Autodesk Fusion 360 part; units mm, degrees
note: some values were not read from the file. Set by a fixed rule: which face or edge a step refers to.
(part 2 of 2)
sketch "Skizze8" plane through (0, 0, 66) normal (0, 0, -1) x (-1, 0, 0)
  circle A0 centre (6.1, 44.01) radius 2
  line L0 (-43.85, 38.01) -> (0.1, 38.01)
  line L1 (0.1, 38.01) -> (0.1, -0.01)
  line L2 (0.1, -0.01) -> (-43.85, -0.01)
  line L3 (-43.85, -0.01) -> (-43.85, 38.01)
  circle A1 centre (-49.85, -6.01) radius 2
  circle A2 centre (-49.85, 44.01) radius 2
  circle A3 centre (6.1, -6.01) radius 2
  arc A4 (-49.85, 48.01) -> (-53.85, 44.01) centre (-49.85, 44.01) ccw
  line L4 (-53.85, 44.01) -> (-53.85, -6.01)
  arc A5 (-53.85, -6.01) -> (-49.85, -10.01) centre (-49.85, -6.01) ccw
  line L5 (-49.85, -10.01) -> (6.1, -10.01)
  arc A6 (6.1, -10.01) -> (10.1, -6.01) centre (6.1, -6.01) ccw
  line L6 (10.1, -6.01) -> (10.1, 44.01)
  arc A7 (10.1, 44.01) -> (6.1, 48.01) centre (6.1, 44.01) ccw
  line L7 (6.1, 48.01) -> (-49.85, 48.01)
  line L8 (0.1, -0.01) -> (-43.85, -0.01)
  line L9 (-43.85, -0.01) -> (-43.85, 38.01)
  line L10 (-43.85, 38.01) -> (0.1, 38.01)
  line L11 (0.1, 38.01) -> (0.1, -0.01)
  line L12 (-43.85, 38.01) -> (0.1, 38.01)
  line L13 (0.1, 38.01) -> (0.1, 38)
  line L14 (0.1, 38) -> (-43.85, 38)
  line L15 (-43.85, 38) -> (-43.85, 38.01)
  line L16 (-43.85, 0) -> (0.1, 0)
  line L17 (0.1, 0) -> (0.1, -0.01)
  line L18 (0.1, -0.01) -> (-43.85, -0.01)
  line L19 (-43.85, -0.01) -> (-43.85, 0)
  line L20 (-43.85, 2) -> (0.1, 2)
  line L21 (0.1, 2) -> (0.1, 0)
  line L22 (0.1, 0) -> (-43.85, 0)
  line L23 (-43.85, 0) -> (-43.85, 2)
  line L24 (-43.85, 4) -> (0.1, 4)
  line L25 (0.1, 4) -> (0.1, 2)
  line L26 (0.1, 2) -> (-43.85, 2)
  line L27 (-43.85, 2) -> (-43.85, 4)
  line L28 (-43.85, 6) -> (0.1, 6)
  line L29 (0.1, 6) -> (0.1, 4)
  line L30 (0.1, 4) -> (-43.85, 4)
  line L31 (-43.85, 4) -> (-43.85, 6)
  line L32 (-43.85, 8) -> (0.1, 8)
  line L33 (0.1, 8) -> (0.1, 6)
  line L34 (0.1, 6) -> (-43.85, 6)
  line L35 (-43.85, 6) -> (-43.85, 8)
  line L36 (-43.85, 10) -> (0.1, 10)
  line L37 (0.1, 10) -> (0.1, 8)
  line L38 (0.1, 8) -> (-43.85, 8)
  line L39 (-43.85, 8) -> (-43.85, 10)
  line L40 (-43.85, 12) -> (0.1, 12)
  line L41 (0.1, 12) -> (0.1, 10)
  line L42 (0.1, 10) -> (-43.85, 10)
  line L43 (-43.85, 10) -> (-43.85, 12)
  line L44 (-43.85, 14) -> (0.1, 14)
  line L45 (0.1, 14) -> (0.1, 12)
  line L46 (0.1, 12) -> (-43.85, 12)
  line L47 (-43.85, 12) -> (-43.85, 14)
  line L48 (-43.85, 16) -> (0.1, 16)
  line L49 (0.1, 16) -> (0.1, 14)
  line L50 (0.1, 14) -> (-43.85, 14)
  line L51 (-43.85, 14) -> (-43.85, 16)
  line L52 (-43.85, 18) -> (0.1, 18)
  line L53 (0.1, 18) -> (0.1, 16)
  line L54 (0.1, 16) -> (-43.85, 16)
  line L55 (-43.85, 16) -> (-43.85, 18)
  line L56 (-43.85, 20) -> (0.1, 20)
  line L57 (0.1, 20) -> (0.1, 18)
  line L58 (0.1, 18) -> (-43.85, 18)
  line L59 (-43.85, 18) -> (-43.85, 20)
  line L60 (-43.85, 22) -> (0.1, 22)
  line L61 (0.1, 22) -> (0.1, 20)
  line L62 (0.1, 20) -> (-43.85, 20)
  line L63 (-43.85, 20) -> (-43.85, 22)
  line L64 (-43.85, 24) -> (0.1, 24)
  line L65 (0.1, 24) -> (0.1, 22)
  line L66 (0.1, 22) -> (-43.85, 22)
  line L67 (-43.85, 22) -> (-43.85, 24)
  line L68 (-43.85, 28) -> (0.1, 28)
  line L69 (0.1, 28) -> (0.1, 26)
  line L70 (0.1, 26) -> (-43.85, 26)
  line L71 (-43.85, 26) -> (-43.85, 28)
  line L72 (-43.85, 26) -> (0.1, 26)
  line L73 (0.1, 26) -> (0.1, 24)
  line L74 (0.1, 24) -> (-43.85, 24)
  line L75 (-43.85, 24) -> (-43.85, 26)
  line L76 (-43.85, 30) -> (0.1, 30)
  line L77 (0.1, 30) -> (0.1, 28)
  line L78 (0.1, 28) -> (-43.85, 28)
  line L79 (-43.85, 28) -> (-43.85, 30)
  line L80 (-43.85, 32) -> (0.1, 32)
  line L81 (0.1, 32) -> (0.1, 30)
  line L82 (0.1, 30) -> (-43.85, 30)
  line L83 (-43.85, 30) -> (-43.85, 32)
  line L84 (-43.85, 34) -> (0.1, 34)
  line L85 (0.1, 34) -> (0.1, 32)
  line L86 (0.1, 32) -> (-43.85, 32)
  line L87 (-43.85, 32) -> (-43.85, 34)
  line L88 (-43.85, 36) -> (0.1, 36)
  line L89 (0.1, 36) -> (0.1, 34)
  line L90 (0.1, 34) -> (-43.85, 34)
  line L91 (-43.85, 34) -> (-43.85, 36)
  line L92 (-43.85, 38) -> (0.1, 38)
  line L93 (0.1, 38) -> (0.1, 36)
  line L94 (0.1, 36) -> (-43.85, 36)
  line L95 (-43.85, 36) -> (-43.85, 38)
  dimension "d154" = 0.01
  dimension "d155" = 0.01
  dimension "d156" = 2
  dimension "d157" = 2
  dimension "d159" = 2
  dimension "d160" = 2
  dimension "d161" = 2
  dimension "d162" = 2
  dimension "d163" = 2
  dimension "d164" = 2
  dimension "d165" = 2
  dimension "d166" = 2
  dimension "d167" = 2
  dimension "d168" = 2
  dimension "d169" = 2
  dimension "d170" = 2
  dimension "d171" = 2
  dimension "d172" = 2
  dimension "d173" = 2
  dimension "d174" = 2
  dimension "d175" = 2
  constraint horizontal L8
  constraint vertical L9
  constraint horizontal L10
  constraint vertical L11
  constraint coincident L0.start L3.end
  constraint coincident L1.end L2.start
  constraint horizontal L12
  constraint vertical L13
  constraint horizontal L14
  constraint vertical L15
  constraint coincident L0.start L15
  constraint coincident L0.start L12
  constraint coincident L0.end L13
  constraint horizontal L16
  constraint vertical L17
  constraint horizontal L18
  constraint vertical L19
  constraint coincident L2.end L19
  constraint coincident L2.end L18
  constraint coincident L1.end L17
  constraint horizontal L20
  constraint vertical L21
  constraint horizontal L22
  constraint vertical L23
  constraint coincident L16.start L23
  constraint coincident L16.start L22
  constraint coincident L16.end L21
  constraint horizontal L24
  constraint vertical L25
  constraint horizontal L26
  constraint vertical L27
  constraint coincident L20.start L26
  constraint coincident L20.start L27
  constraint coincident L20.end L25
  constraint horizontal L28
  constraint vertical L29
  constraint horizontal L30
  constraint vertical L31
  constraint coincident L24.start L30
  constraint coincident L24.start L31
  constraint coincident L24.end L29
  constraint horizontal L32
  constraint vertical L33
  constraint horizontal L34
  constraint vertical L35
  constraint coincident L28.start L34
  constraint coincident L28.start L35
  constraint coincident L28.end L33
  constraint horizontal L36
  constraint vertical L37
  constraint horizontal L38
  constraint vertical L39
  constraint coincident L32.start L38
  constraint coincident L32.start L39
  constraint coincident L32.end L37
  constraint horizontal L40
  constraint vertical L41
  constraint horizontal L42
  constraint vertical L43
  constraint coincident L36.start L42
  constraint coincident L36.start L43
  constraint coincident L36.end L41
  constraint horizontal L44
  constraint vertical L45
  constraint horizontal L46
  constraint vertical L47
  constraint coincident L40.start L46
  constraint coincident L40.start L47
  constraint coincident L40.end L45
  constraint horizontal L48
  constraint vertical L49
  constraint horizontal L50
  constraint vertical L51
  constraint coincident L44.start L50
  constraint coincident L44.start L51
  constraint coincident L44.end L49
  constraint horizontal L52
  constraint vertical L53
  constraint horizontal L54
  constraint vertical L55
  constraint horizontal L56
  constraint vertical L57
  constraint horizontal L58
  constraint vertical L59
  constraint horizontal L60
  constraint vertical L61
  constraint horizontal L62
  constraint vertical L63
  constraint coincident L48.start L54
  constraint coincident L48.start L55
  constraint coincident L48.end L53
  constraint coincident L52.start L58
  constraint coincident L52.start L59
  constraint coincident L52.end L57
  constraint horizontal L64
  constraint vertical L65
  constraint horizontal L66
  constraint vertical L67
  constraint coincident L56.start L62
  constraint coincident L56.start L63
  constraint coincident L56.end L61
  constraint coincident L60.start L66
  constraint coincident L60.start L67
  constraint coincident L60.end L65
  constraint horizontal L68
  constraint vertical L69
  constraint horizontal L70
  constraint vertical L71
  constraint horizontal L72
  constraint vertical L73
  constraint horizontal L74
  constraint vertical L75
  constraint coincident L64.start L74
  constraint coincident L64.start L75
  constraint coincident L64.end L73
  constraint coincident L70 L71.start
  constraint coincident L71 L70.end
  constraint coincident L69 L70.start
  constraint horizontal L76
  constraint vertical L77
  constraint horizontal L78
  constraint vertical L79
  constraint horizontal L80
  constraint vertical L81
  constraint horizontal L82
  constraint vertical L83
  constraint coincident L68.start L78
  constraint coincident L68.start L79
  constraint coincident L68.end L77
  constraint coincident L76.start L82
  constraint coincident L76.start L83
  constraint coincident L76.end L81
  constraint horizontal L84
  constraint vertical L85
  constraint horizontal L86
  constraint vertical L87
  constraint horizontal L88
  constraint vertical L89
  constraint horizontal L90
  constraint vertical L91
  constraint coincident L80.start L86
  constraint coincident L80.start L87
  constraint coincident L80.end L85
  constraint coincident L84.start L90
  constraint coincident L84.start L91
  constraint coincident L84.end L89
  constraint horizontal L92
  constraint vertical L93
  constraint horizontal L94
  constraint vertical L95
  constraint coincident L88.start L94
  constraint coincident L88.start L95
  constraint coincident L88.end L93
  measures "d154" distance of L0.start L14.end
  measures "d155" distance of L16.start L2.end
  measures "d156" distance of L20.start L16.start
  measures "d157" distance of L24.start L20.start
  measures "d159" distance of L28.start L24.start
  measures "d160" distance of L32.start L28.start
  measures "d161" distance of L36.start L32.start
  measures "d162" distance of L40.start L36.start
  measures "d163" distance of L44.start L40.start
  measures "d164" distance of L48.start L44.start
  measures "d165" distance of L52.start L48.start
  measures "d166" distance of L56.start L52.start
  measures "d167" distance of L60.start L56.start
  measures "d168" distance of L64.start L60.start
  measures "d169" distance of L70.end L64.start
  measures "d170" distance of L68.start L70.end
  measures "d171" distance of L76.start L68.start
  measures "d172" distance of L80.start L76.start
  measures "d173" distance of L84.start L80.start
  measures "d174" distance of L88.start L84.start
  measures "d175" distance of L14.end L88.start
extrude "Extrusion21" add sketch "Skizze8" against normal blind 4 contours L0 L1 L3 L9 L10 L11 L12 L13 L14 L15 L92 | L1 L3 L9 L11 L84 L88 L89 L90 L91 L94 | L1 L3 L9 L11 L76 L80 L81 L82 L83 L86 | L1 L3 L9 L11 L68 L69 L70 L71 L72 L78 | L1 L3 L9 L11 L60 L64 L65 L66 L67 L74 | L1 L3 L9 L11 L52 L56 L57 L58 L59 L62 | L1 L3 L9 L11 L44 L48 L49 L50 L51 L54 | L1 L3 L9 L11 L36 L40 L41 L42 L43 L46 | L1 L3 L9 L11 L28 L32 L33 L34 L35 L38 | L1 L3 L9 L11 L20 L24 L25 L26 L27 L30 | L1 L2 L3 L8 L9 L11 L16 L17 L18 L19 L22 bodies 2
copy_body "Körper kopieren/einfügen25" bodies 5 makes body 17
copy_body "Körper kopieren/einfügen26" bodies 5 makes body 18
move_body "Verschieben28" bodies 18 to x (1, 0, 0) y (0, 1, 0) z (0, 0, 1) at (0, 0, 4)
hidden bodies 3 4 7 17 18
equation "d1 = d2 * 0.625"
equation "d15 = d2 / 3"
equation "d16 = d15"
equation "d17 = d1 / 8"
equation "d22 = d21"
equation "d23 = d130"
equation "d24 = d23"
equation "d25 = d28"
equation "d26 = d24"
equation "d27 = d1 / 1 / 5"
equation "d28 = d1 * 1 / 5"
equation "d29 = d26"
equation "d30 = d27"
equation "d31 = d24"
equation "d32 = d34"
equation "d37 = d23"
equation "d38 = d31"
equation "d39 = 2 mm"
equation "d42 = ( d39 * 10 ) + ( 9 * d126 ) + 2 * d41"
equation "d44 = d43"
equation "d46 = d45"
equation "d48 = d47"
equation "d50 = d49"
equation "d51 = d49"
equation "d52 = d49"
equation "d57 = d130"
equation "d59 = -d36 - 0.5 mm"
equation "d61 = -d36 - 0.5 mm"
equation "d64 = d63"
equation "d65 = d63"
equation "d66 = d63"
equation "d67 = d65"
equation "d68 = d63"
equation "d69 = d42"
equation "d73 = -d39"
equation "d75 = -d130"
equation "d77 = d39 + d41"
equation "d78 = d41"
equation "d79 = d41"
equation "d80 = d39"
equation "d81 = d80"
equation "d82 = d126"
equation "d83 = d80"
equation "d84 = d82"
equation "d85 = d83"
equation "d86 = d84"
equation "d87 = d85"
equation "d88 = d86"
equation "d89 = d87"
equation "d90 = d88"
equation "d91 = d79"
equation "d92 = d126"
equation "d93 = d81"
equation "d94 = d92"
equation "d95 = d93"
equation "d96 = d94"
equation "d97 = d95"
equation "d98 = d96"
equation "d99 = d97"
equation "d100 = d98"
equation "d101 = d78"
equation "d132 = d89"
equation "d133 = d90"
equation "d134 = d132"
equation "d135 = d133"
equation "d136 = d99"
equation "d137 = d100"
equation "d138 = d136"
equation "d139 = d137"
equation "d140 = d134"
equation "d141 = d135"
equation "d142 = d140"
equation "d143 = d141"
equation "d144 = d142"
equation "d146 = d138"
equation "d147 = d139"
equation "d148 = d146"
equation "d149 = d147"
equation "d150 = d148"
equation "d151 = -d130"
equation "d154 = d78"
equation "d155 = d78"
equation "d156 = d39"
equation "d157 = d126"
equation "d159 = d156"
equation "d160 = d157"
equation "d161 = d159"
equation "d162 = d160"
equation "d163 = d161"
equation "d164 = d162"
equation "d165 = d163"
equation "d166 = d164"
equation "d167 = d165"
equation "d168 = d166"
equation "d169 = d167"
equation "d170 = d168"
equation "d171 = d169"
equation "d172 = d170"
equation "d173 = d171"
equation "d174 = d172"
equation "d175 = d173"
equation "d176 = -d130"
named bodies: "number_0", "0_top_cover", "1_top_mount", "5_bottom", "4_pcb", "2_lightguide_top", "3_lightguide_bottom", "number_0 (1)", "number_0 (1) (1)", "number_0 (1) (1) (1)", "number_0 (1) (1) (1) (1)", "number_0 (1) (1) (1) (1) (1)", "number_0 (1) (1) (1) (1) (1) (1)", "number_0 (1) (1) (1) (1) (1) (1) (1)", "number_0 (1) (1) (1) (1) (1) (1) (1) (1)", "number_0 (1) (1) (1) (1) (1) (1) (1) (1) (1)", "4_pcb (1)", "4_pcb (1) (1)"
